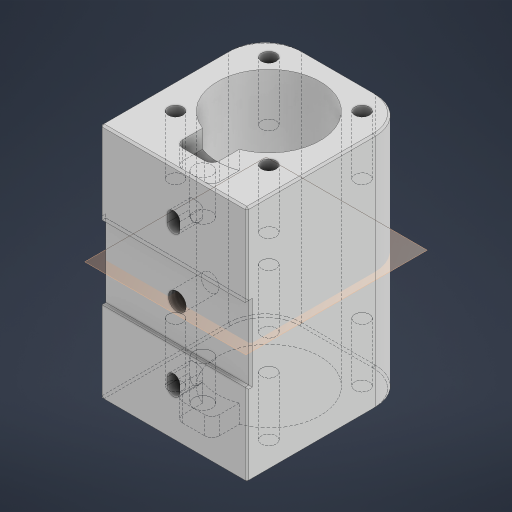
# Autodesk Inventor part: sf_Cylinder_1
Saved by Autodesk Inventor 2024 (Build 280153000, 153)
## iProperties
Created: 2024-03-20
Part Number: sf_Cylinder_1
Material: Generisch
Document SubType Name: Modeling
Designer: Simon
Density: 1 g/cm^3
Appearance: Vorgabe
Author: Simon
Autodesk Inventor part; units mm, degrees
ref_plane "YZ Plane" through (0, 0, 0) normal (1, 0, 0) x (0, 1, 0)
ref_plane "XZ Plane" through (0, 0, 0) normal (0, 1, 0) x (-1, 0, 0)
ref_plane "XY Plane" through (0, 0, 0) normal (0, 0, 1) x (1, 0, 0)
sketch "Skizze1" plane through (0, 0, 0) normal (0, 0, 1) x (1, 0, 0)
  circle A0 centre (0, 3.5) radius 14
  line L0 (-20, -22.5) -> (20, -22.5)
  line L1 (20, -22.5) -> (20, 12.5)
  line L2 (10, 22.5) -> (-10, 22.5)
  line L3 (-20, 12.5) -> (-20, -22.5)
  arc A1 (-10, 22.5) -> (-20, 12.5) centre (-10, 12.5) ccw
  arc A2 (20, 12.5) -> (10, 22.5) centre (10, 12.5) ccw
  dimension "d0" = 28
  dimension "d3" = 10
  dimension "d13" = 19
  constraints: 8 end point, 4 point on circle, 4 tangent, 3 centre point, 2 parallel, 1 equal radius, 1 horizontal, 1 perpendicular
  measures "d0" diameter of A0
  measures "d3" radius of A1
  measures "d13" distance from line of L2 A0.centre
extrude "Extrusion1" add sketch "Skizze1" along normal mid plane 65
sketch "Skizze2" plane through (0, 0, 32.5) normal (0, 0, 1) x (1, 0, 0)
  circle A0 centre (0, 3.5) radius 18 construction
  circle A1 centre (0, -14.5) radius 2.5
  line L0 (-18, -14.5) -> (18, -14.5)
  line L1 (18, -14.5) -> (18, 21.5)
  line L2 (18, 21.5) -> (-18, 21.5)
  line L3 (-18, 21.5) -> (-18, -14.5)
  line L4 (-18, -14.5) -> (18, 21.5) construction
  line L5 (18, -14.5) -> (-18, 21.5) construction
  circle A2 centre (12.7279, 16.2279) radius 2
  circle A3 centre (12.7279, -9.2279) radius 2
  circle A4 centre (-12.7279, -9.2279) radius 2
  circle A5 centre (-12.7279, 16.2279) radius 2
  circle A6 centre (0, 3.5) radius 14
  dimension "d6" = 36
  dimension "d7" = 5
  dimension "d8" = 4
  dimension "d9" = 4
  dimension "d10" = 4
  dimension "d11" = 4
  constraints: 12 end point, 7 centre point, 5 point on circle, 4 point on line, 2 midpoint, 1 coincident
  measures "d6" diameter of A0
  measures "d7" diameter of A1
  measures "d8" diameter of A2
  measures "d9" diameter of A3
  measures "d10" diameter of A4
  measures "d11" diameter of A5
extrude "Extrusion2" cut sketch "Skizze2" against normal blind 16 contours L0 A1 | A1 L0 | A2 | A3 | A4 | A5
sketch "Skizze3" plane through (0, 0, 32.5) normal (0, 0, 1) x (1, 0, 0)
  line L0 (-3, -17) -> (3, -17)
  line L1 (5, -15) -> (5, -12)
  line L2 (5, -12) -> (-5, -12)
  line L3 (-5, -12) -> (-5, -15)
  circle A0 centre (0, -14.5) radius 2.5 projected
  line L4 (-5, -17) -> (5, -12) construction
  line L5 (5, -17) -> (-5, -12) construction
  circle A1 centre (0, 3.5) radius 14 projected
  line L6 (-5, -12) -> (5, -12)
  line L7 (5, -12) -> (5, -9.5767)
  line L8 (5, -9.5767) -> (-5, -9.5767)
  line L9 (-5, -9.5767) -> (-5, -12)
  arc A2 (-5, -15) -> (-3, -17) centre (-3, -15) ccw
  arc A3 (3, -17) -> (5, -15) centre (3, -15) ccw
  point P0 (0, 0)
  dimension "d16" = 10
  dimension "d17" = 2
  constraints: 20 end point, 4 parallel, 4 point on circle, 4 point on line, 4 tangent, 2 centre point, 2 horizontal, 2 midpoint, 2 perpendicular, 1 equal radius, 2 other
  measures "d16" distance of L2.end L1.end
  measures "d17" radius of A2
extrude "Extrusion3" cut sketch "Skizze3" against normal blind 5 contours A2 L3 L2 A0 L0 | A0 L2 L1 A3 L0 | A0 | L2 L9 A1 L7
sketch "Skizze4" plane through (-20, -22.5, 32.5) normal (0, -1, 0) x (1, 0, 0)
  line L0 (17.5, -16) -> (22.5, -16) projected
  line L1 (17.5, -5) -> (17.5, -16) projected
  line L2 (22.5, -5) -> (22.5, -16) projected
  line L3 (17.5, -16) -> (22.5, -16)
  line L4 (22.5, -16) -> (22.5, -10.5)
  line L5 (22.5, -10.5) -> (17.5, -10.5)
  line L6 (17.5, -10.5) -> (17.5, -16)
  line L7 (20, -16) -> (20, -10.5) construction
  line L8 (21.75, -14.25) -> (21.75, -12.25)
  line L9 (18.25, -12.25) -> (18.25, -14.25)
  arc A0 (18.25, -14.25) -> (21.75, -14.25) centre (20, -14.25) ccw
  arc A1 (21.75, -12.25) -> (18.25, -12.25) centre (20, -12.25) ccw
  point P0 (20, -32.5)
  point P1 (20, -13.25)
  dimension "d20" = 5.5
  dimension "d21" = 3.5
  constraints: 16 end point, 6 point on circle, 4 midpoint, 4 tangent, 3 parallel, 2 centre point, 2 point on line, 1 horizontal, 1 perpendicular
  measures "d20" distance of L4.end L3.end
  measures "d21" diameter of A1
extrude "Extrusion4" cut sketch "Skizze4" against normal up to surface contours A0 L9 A1 L8
sketch "Skizze5" plane through (-20, -22.5, 32.5) normal (0, -1, 0) x (1, 0, 0)
  line L0 (40, 0) -> (40, -65) projected
  line L1 (0, -22.5) -> (40, -22.5)
  line L2 (40, -22.5) -> (40, -42.5)
  line L3 (40, -42.5) -> (0, -42.5)
  line L4 (0, -42.5) -> (0, -22.5)
  line L5 (0, -22.5) -> (40, -42.5) construction
  line L6 (40, -22.5) -> (0, -42.5) construction
  point P0 (20, -32.5)
  dimension "d24" = 20
  constraints: 12 end point, 2 midpoint, 2 parallel, 1 horizontal, 1 perpendicular, 1 point on line
  measures "d24" distance of L1.end L2.end
extrude "Extrusion5" cut sketch "Skizze5" against normal blind 1
sketch "Skizze6" plane through (-20, -21.5, 32.5) normal (0, -1, 0) x (1, 0, 0)
  point P0 (20, -32.5)
hole "Bohrung1" at (0, -21.5, 0) direction (0, 1, 0) diameter 4.917 depth 9 thread size "M6x1" class "6H" standard "ISO Metric profile"
ref_plane "Arbeitsebene1" through (0, 0, 0) normal (0, 0, 1) x (1, 0, 0)
mirror "Spiegeln1" about plane through (0, 0, 0) normal (0, 0, 1) of "Extrusion3", "Extrusion2", "Extrusion4"
chamfer "Fasen1" distance 0.5 angle 45 22 edges at (20, -5, 32.5) (17.0711, 19.5711, 32.5) (0, 22.5, 32.5) (-17.0711, 19.5711, 32.5) (-20, -5, 32.5) (20, -22.5, 21.25) (20, -21.5, 0) (20, -22.5, -21.25) (0, -22.5, 32.5) (-20, -22.5, 21.25) (-20, -22.5, -21.25) (17.0711, 19.5711, -32.5) (20, -5, -32.5) (0, 22.5, -32.5) (-17.0711, 19.5711, -32.5) (-20, -5, -32.5) (-20, -21.5, 0) (-20, -22, 10) (-20, -22, -10) (20, -22, -10) (20, -22, 10) (0, -22.5, -32.5)
